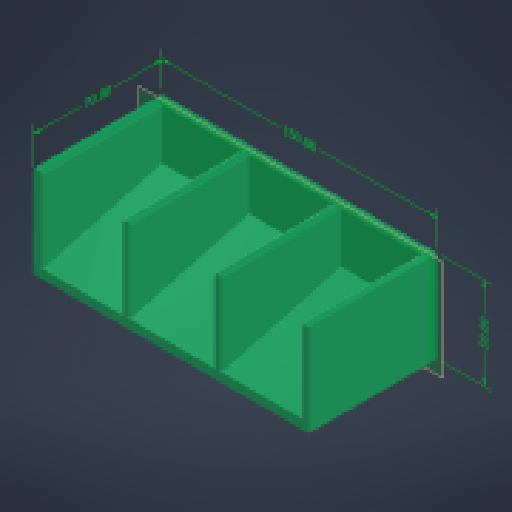
# Autodesk Inventor part: rubbish-container-group2
Saved by Autodesk Inventor 2026.2 (Build 302298010, 298A)
## iProperties
Created: 2026-02-23
Part Number: rubbish-container-group2
Material: ABS Plastic
Document SubType Name: Modeling
Designer: ts2104
Density: 1.06 g/cm^3
Appearance: Smooth - White
Author: ts2104
Autodesk Inventor part; units mm, degrees
ref_plane "YZ Plane" through (0, 0, 0) normal (1, 0, 0) x (0, 1, 0)
ref_plane "XZ Plane" through (0, 0, 0) normal (0, 1, 0) x (-1, 0, 0)
ref_plane "XY Plane" through (0, 0, 0) normal (0, 0, 1) x (1, 0, 0)
sketch "Sketch1" plane through (0, 0, 0) normal (0, 0, 1) x (1, 0, 0)
  line L0 (-75, 25) -> (75, 25)
  line L1 (75, 25) -> (75, -25)
  line L2 (75, -25) -> (-75, -25)
  line L3 (-75, -25) -> (-75, 25)
  line L4 (-75, 25) -> (75, -25) construction
  line L5 (75, 25) -> (-75, -25) construction
  line L6 (25, 25) -> (25, -25)
  line L7 (22.5, 25) -> (27.5, 25)
  line L8 (27.5, 25) -> (27.5, -25)
  line L9 (27.5, -25) -> (22.5, -25)
  line L10 (22.5, -25) -> (22.5, 25)
  line L11 (22.5, 25) -> (27.5, -25) construction
  line L12 (27.5, 25) -> (22.5, -25) construction
  line L13 (75, 25) -> (70, 25)
  line L14 (70, 25) -> (70, -25)
  line L15 (70, -25) -> (75, -25)
  line L16 (75, -25) -> (75, 25)
  point P0 (0, 0)
  point P1 (25, 0)
  point P2 (22.5, 25)
  point P3 (22.5, -25)
  point P4 (27.5, -25)
  point P5 (27.5, 25)
  dimension "d0" = 50
  dimension "d1" = 150
  dimension "d9" = 50
  dimension "d14" = 5
  dimension "d15" = 5
  constraints: 34 end point, 6 parallel, 5 midpoint, 4 perpendicular, 3 horizontal, 2 collinear, 2 point on line
  measures "d0" distance of L2.end L0.start
  measures "d1" distance of L0.start L0.end
  measures "d9" distance between parallel lines of L6 L1
  measures "d14" distance of L8.end L9.end
  measures "d15" distance of L15.end L14.end
sketch "Sketch2" plane through (0, 0, 0) normal (1, 0, 0) x (0, 1, 0)
  line L0 (25, 0) -> (-25, 0) projected
  line L1 (25, 0) -> (-25, 0)
  line L2 (-25, 0) -> (-25, 70)
  line L3 (-25, 70) -> (25, 70)
  line L4 (25, 70) -> (25, 0)
  line L5 (-20, 70) -> (-1.2436, 0)
  line L6 (25, 5) -> (-25, 5)
  line L7 (-20, 70) -> (-20, 0)
  point P0 (0, 0)
  point P1 (-1.2436, 0)
  point P2 (-2.5833, 5)
  dimension "d2" = 70
  dimension "d3" = 5
  dimension "d5" = 5
  dimension "d20" = 15
  constraints: 14 end point, 5 point on line, 3 equal length, 3 perpendicular
  measures "d2" distance of L0.end L2.end
  measures "d3" distance of L2.end L5.start
  measures "d5" distance between parallel lines of L0 L6
  measures "d20" angle of L7 L5
extrude "Extrusion1" add sketch "Sketch2" along normal blind 75 contours L0 L7 L6 L5 | L0 L2 L6 L7 | L6 L7 L5 | L6 L2 L3 L7
extrude "Extrusion2" add sketch "Sketch2" along normal blind 75 contours L0 L5 L6 L4
extrude "Extrusion3" add sketch "Sketch1" along normal blind 70 contours L0 L1 L2 L14
extrude "Extrusion4" add sketch "Sketch1" along normal blind 70 contours L0 L6 L2 L10 | L0 L8 L2 L6
mirror "Mirror1" about plane through (0, 0, 0) normal (1, 0, 0)
fillet "Fillet1" radius 2 9 edges at (-27.5, 25, 37.5) (-22.5, 25, 37.5) (22.5, 25, 37.5) (27.5, 25, 37.5) (70, 25, 37.5) (-70, 25, 37.5) (-48.75, 25, 5) (0, 25, 5) (48.75, 25, 5)
fillet "Fillet2" radius 2 16 edges at (-26.9142, 24.4142, 70) (-25, 25, 70) (-23.0858, 24.4142, 70) (-22.5, 1.5, 70) (-27.5, 1.5, 70) (23.0858, 24.4142, 70) (25, 25, 70) (26.9142, 24.4142, 70) (27.5, 1.5, 70) (22.5, 1.5, 70) (70.5858, 24.4142, 70) (73.5, 25, 70) (70, 1.5, 70) (-70.5858, 24.4142, 70) (-73.5, 25, 70) (-70, 1.5, 70)
sketch "Sketch3" plane through (75, -25, 0) normal (0, -1, 0) x (1, 0, 0)
  line L0 (0, 0) -> (-150, 0) projected
  line L1 (0, 70) -> (0, 0) projected
  line L2 (-150, 70) -> (0, 70) projected
  line L3 (-150, 70) -> (-150, 0) projected
  line L4 (-145, 5) -> (-5, 5)
  line L5 (-5, 5) -> (-5, 65)
  line L6 (-5, 65) -> (-145, 65)
  line L7 (-145, 65) -> (-145, 5)
  circle A0 centre (-5, 5) radius 2.2
  circle A1 centre (-145, 5) radius 2.2
  point P0 (-75, 0)
  dimension "d35" = 5
  dimension "d36" = 4.4
  dimension "d37" = 4.4
  constraints: 8 end point, 2 centre point, 2 coincident, 3 other
  measures "d35" distance between parallel lines of L0 L4
  measures "d36" diameter of A0
  measures "d37" diameter of A1
extrude "Extrusion5" cut sketch "Sketch3" against normal blind 10 contours L7 A1 L4 | L4 A1 L7 | A0 L5 L4 | L4 L5 A0
fillet "Fillet3" radius 1 2 edges at (67.8, -25, 5) (-72.2, -25, 5)
ref_plane "Work Plane2" through (75, -25, 5) normal (0, 0, -1) x (-1, 0, 0)
fillet "Fillet4" radius 1 1 edges at (-72.2, -15, 5)
fillet "Fillet5" radius 1 1 edges at (67.8, -15, 5)
equation "\"d9\" = 0.333333 * d1"
equation "\"d5\" = d3"
equation "\"d10\" = 0.5 * d1"
equation "\"d12\" = 0.5 * d1"
equation "\"d16\" = d2"
equation "\"d18\" = d2"
body "Solid1"
